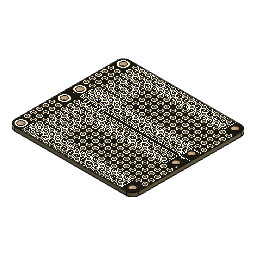
2890 Doubler FeatherWing (Autodesk Fusion 360 design; units mm, degrees)
part number: FEATHERWING_NODIM
Autodesk Fusion 360 part; units mm, degrees
sketch "sketch 305" plane through (0, 0, 0) normal (0, 0, 1) x (1, 0, 0)
  line L0 (2.54, 46.99) -> (48.26, 46.99)
  arc A0 (50.8, 44.45) -> (48.26, 46.99) centre (48.26, 44.45) ccw
  line L1 (50.8, 44.45) -> (50.8, 2.54)
  arc A1 (48.26, 0) -> (50.8, 2.54) centre (48.26, 2.54) ccw
  line L2 (48.26, 0) -> (2.54, 0)
  arc A2 (0, 2.54) -> (2.54, 0) centre (2.54, 2.54) ccw
  line L3 (0, 2.54) -> (0, 44.45)
  arc A3 (2.54, 46.99) -> (0, 44.45) centre (2.54, 44.45) ccw
extrude "Board" add sketch "sketch 305" along normal blind 1.57 makes body 1 in component "Board"
sketch "sketch 2573" plane through (0, 0, 0) normal (0, 0, 1) x (1, 0, 0)
  line L0 (0, 0) -> (50.8, 0)
  line L1 (50.8, 0) -> (50.8, 22.86)
  line L2 (50.8, 22.86) -> (0, 22.86)
  line L3 (0, 22.86) -> (0, 0)
extrude "FEATHERWING_DIM" add sketch "sketch 2573" along normal blind 0.1 separate body makes body 2 in component "FEATHERWING_DIM"
sketch "sketch 2713" plane through (0, 0, 0) normal (0, 0, 1) x (1, 0, 0)
  line L0 (-19.55, -0.5) -> (19.55, -0.5)
  line L1 (19.55, -0.5) -> (19.55, 0.5)
  line L2 (19.55, 0.5) -> (-19.55, 0.5)
  line L3 (-19.55, 0.5) -> (-19.55, -0.5)
extrude "1X16_ROUND_76MIL" add sketch "sketch 2713" along normal blind 0.1 separate body makes body 3 in component "1X16_ROUND_76MIL"
sketch "sketch 2853" plane through (0, 0, 0) normal (0, 0, 1) x (1, 0, 0)
  line L0 (-15.24, -0.635) -> (14.47, -0.635)
  line L1 (14.47, -0.635) -> (14.47, 0.635)
  line L2 (14.47, 0.635) -> (-15.24, 0.635)
  line L3 (-15.24, 0.635) -> (-15.24, -0.635)
extrude "1X12_ROUND_76MIL" add sketch "sketch 2853" along normal blind 0.1 separate body makes body 4 in component "1X12_ROUND_76MIL"
sketch "sketch 437" plane through (0, 0, 0) normal (0, 0, 1) x (1, 0, 0)
  circle A0 centre (13.97, 6.35) radius 0.55
  circle A1 centre (13.97, 8.89) radius 0.55
  circle A2 centre (13.97, 11.43) radius 0.55
  circle A3 centre (13.97, 13.97) radius 0.55
  circle A4 centre (13.97, 16.51) radius 0.55
  circle A5 centre (13.97, 19.05) radius 0.55
  circle A6 centre (13.97, 21.59) radius 0.55
  circle A7 centre (13.97, 45.72) radius 0.55
  circle A8 centre (13.97, 43.18) radius 0.55
  circle A9 centre (13.97, 40.64) radius 0.55
  circle A10 centre (13.97, 38.1) radius 0.55
  circle A11 centre (13.97, 35.56) radius 0.55
  circle A12 centre (13.97, 33.02) radius 0.55
  circle A13 centre (13.97, 30.48) radius 0.55
  circle A14 centre (8.89, 6.35) radius 0.55
  circle A15 centre (8.89, 8.89) radius 0.55
  circle A16 centre (8.89, 11.43) radius 0.55
  circle A17 centre (8.89, 13.97) radius 0.55
  circle A18 centre (8.89, 16.51) radius 0.55
  circle A19 centre (8.89, 19.05) radius 0.55
  circle A20 centre (8.89, 21.59) radius 0.55
  circle A21 centre (8.89, 30.48) radius 0.55
  circle A22 centre (8.89, 33.02) radius 0.55
  circle A23 centre (8.89, 35.56) radius 0.55
  circle A24 centre (8.89, 38.1) radius 0.55
  circle A25 centre (8.89, 40.64) radius 0.55
  circle A26 centre (8.89, 43.18) radius 0.55
  circle A27 centre (8.89, 45.72) radius 0.55
  circle A28 centre (6.35, 6.35) radius 0.55
  circle A29 centre (11.43, 6.35) radius 0.55
  circle A30 centre (11.43, 8.89) radius 0.55
  circle A31 centre (6.35, 8.89) radius 0.55
  circle A32 centre (6.35, 11.43) radius 0.55
  circle A33 centre (3.81, 6.35) radius 0.55
  circle A34 centre (1.27, 6.35) radius 0.55
  circle A35 centre (1.27, 8.89) radius 0.55
  circle A36 centre (3.81, 8.89) radius 0.55
  circle A37 centre (3.81, 11.43) radius 0.55
  circle A38 centre (1.27, 11.43) radius 0.55
  circle A39 centre (1.27, 13.97) radius 0.55
  circle A40 centre (3.81, 13.97) radius 0.55
  circle A41 centre (6.35, 13.97) radius 0.55
  circle A42 centre (11.43, 13.97) radius 0.55
  circle A43 centre (11.43, 11.43) radius 0.55
  circle A44 centre (1.27, 16.51) radius 0.55
  circle A45 centre (3.81, 16.51) radius 0.55
  circle A46 centre (6.35, 16.51) radius 0.55
  circle A47 centre (11.43, 16.51) radius 0.55
  circle A48 centre (11.43, 21.59) radius 0.55
  circle A49 centre (11.43, 19.05) radius 0.55
  circle A50 centre (6.35, 21.59) radius 0.55
  circle A51 centre (6.35, 19.05) radius 0.55
  circle A52 centre (16.51, 6.35) radius 0.55
  circle A53 centre (16.51, 8.89) radius 0.55
  circle A54 centre (16.51, 11.43) radius 0.55
  circle A55 centre (16.51, 13.97) radius 0.55
  circle A56 centre (16.51, 16.51) radius 0.55
  circle A57 centre (19.05, 16.51) radius 0.55
  circle A58 centre (19.05, 13.97) radius 0.55
  circle A59 centre (19.05, 11.43) radius 0.55
  circle A60 centre (19.05, 8.89) radius 0.55
  circle A61 centre (19.05, 6.35) radius 0.55
  circle A62 centre (21.59, 6.35) radius 0.55
  circle A63 centre (21.59, 8.89) radius 0.55
  circle A64 centre (21.59, 11.43) radius 0.55
  circle A65 centre (21.59, 13.97) radius 0.55
  circle A66 centre (21.59, 16.51) radius 0.55
  circle A67 centre (24.13, 16.51) radius 0.55
  circle A68 centre (24.13, 13.97) radius 0.55
  circle A69 centre (24.13, 11.43) radius 0.55
  circle A70 centre (24.13, 8.89) radius 0.55
  circle A71 centre (24.13, 6.35) radius 0.55
  circle A72 centre (26.67, 6.35) radius 0.55
  circle A73 centre (26.67, 8.89) radius 0.55
  circle A74 centre (26.67, 11.43) radius 0.55
  circle A75 centre (26.67, 13.97) radius 0.55
  circle A76 centre (26.67, 16.51) radius 0.55
  circle A77 centre (29.21, 16.51) radius 0.55
  circle A78 centre (29.21, 13.97) radius 0.55
  circle A79 centre (29.21, 11.43) radius 0.55
  circle A80 centre (29.21, 8.89) radius 0.55
  circle A81 centre (29.21, 6.35) radius 0.55
  circle A82 centre (31.75, 6.35) radius 0.55
  circle A83 centre (34.29, 6.35) radius 0.55
  circle A84 centre (36.83, 6.35) radius 0.55
  circle A85 centre (39.37, 6.35) radius 0.55
  circle A86 centre (41.91, 6.35) radius 0.55
  circle A87 centre (41.91, 8.89) radius 0.55
  circle A88 centre (41.91, 11.43) radius 0.55
  circle A89 centre (41.91, 13.97) radius 0.55
  circle A90 centre (41.91, 16.51) radius 0.55
  circle A91 centre (39.37, 16.51) radius 0.55
  circle A92 centre (39.37, 13.97) radius 0.55
  circle A93 centre (39.37, 11.43) radius 0.55
  circle A94 centre (39.37, 8.89) radius 0.55
  circle A95 centre (36.83, 8.89) radius 0.55
  circle A96 centre (36.83, 11.43) radius 0.55
  circle A97 centre (36.83, 13.97) radius 0.55
  circle A98 centre (36.83, 16.51) radius 0.55
  circle A99 centre (34.29, 16.51) radius 0.55
  circle A100 centre (34.29, 13.97) radius 0.55
  circle A101 centre (34.29, 11.43) radius 0.55
  circle A102 centre (34.29, 8.89) radius 0.55
  circle A103 centre (31.75, 8.89) radius 0.55
  circle A104 centre (31.75, 11.43) radius 0.55
  circle A105 centre (31.75, 13.97) radius 0.55
  circle A106 centre (31.75, 16.51) radius 0.55
  circle A107 centre (44.45, 16.51) radius 0.55
  circle A108 centre (44.45, 13.97) radius 0.55
  circle A109 centre (44.45, 11.43) radius 0.55
  circle A110 centre (44.45, 8.89) radius 0.55
  circle A111 centre (44.45, 6.35) radius 0.55
  circle A112 centre (46.99, 6.35) radius 0.55
  circle A113 centre (49.53, 6.35) radius 0.55
  circle A114 centre (49.53, 8.89) radius 0.55
  circle A115 centre (46.99, 8.89) radius 0.55
  circle A116 centre (46.99, 11.43) radius 0.55
  circle A117 centre (49.53, 11.43) radius 0.55
  circle A118 centre (49.53, 13.97) radius 0.55
  circle A119 centre (46.99, 13.97) radius 0.55
  circle A120 centre (46.99, 16.51) radius 0.55
  circle A121 centre (49.53, 16.51) radius 0.55
  circle A122 centre (44.45, 30.48) radius 0.55
  circle A123 centre (44.45, 33.02) radius 0.55
  circle A124 centre (44.45, 35.56) radius 0.55
  circle A125 centre (44.45, 38.1) radius 0.55
  circle A126 centre (44.45, 40.64) radius 0.55
  circle A127 centre (41.91, 40.64) radius 0.55
  circle A128 centre (41.91, 38.1) radius 0.55
  circle A129 centre (41.91, 35.56) radius 0.55
  circle A130 centre (41.91, 33.02) radius 0.55
  circle A131 centre (41.91, 30.48) radius 0.55
  circle A132 centre (46.99, 30.48) radius 0.55
  circle A133 centre (46.99, 33.02) radius 0.55
  circle A134 centre (46.99, 35.56) radius 0.55
  circle A135 centre (46.99, 38.1) radius 0.55
  circle A136 centre (46.99, 40.64) radius 0.55
  circle A137 centre (49.53, 40.64) radius 0.55
  circle A138 centre (49.53, 38.1) radius 0.55
  circle A139 centre (49.53, 35.56) radius 0.55
  circle A140 centre (49.53, 33.02) radius 0.55
  circle A141 centre (49.53, 30.48) radius 0.55
  circle A142 centre (39.37, 30.48) radius 0.55
  circle A143 centre (39.37, 33.02) radius 0.55
  circle A144 centre (39.37, 35.56) radius 0.55
  circle A145 centre (39.37, 38.1) radius 0.55
  circle A146 centre (39.37, 40.64) radius 0.55
  circle A147 centre (36.83, 40.64) radius 0.55
  circle A148 centre (36.83, 38.1) radius 0.55
  circle A149 centre (36.83, 35.56) radius 0.55
  circle A150 centre (36.83, 33.02) radius 0.55
  circle A151 centre (36.83, 30.48) radius 0.55
  circle A152 centre (34.29, 30.48) radius 0.55
  circle A153 centre (34.29, 33.02) radius 0.55
  circle A154 centre (34.29, 35.56) radius 0.55
  circle A155 centre (34.29, 38.1) radius 0.55
  circle A156 centre (34.29, 40.64) radius 0.55
  circle A157 centre (31.75, 40.64) radius 0.55
  circle A158 centre (31.75, 38.1) radius 0.55
  circle A159 centre (31.75, 35.56) radius 0.55
  circle A160 centre (31.75, 33.02) radius 0.55
  circle A161 centre (31.75, 30.48) radius 0.55
  circle A162 centre (29.21, 30.48) radius 0.55
  circle A163 centre (29.21, 33.02) radius 0.55
  circle A164 centre (29.21, 35.56) radius 0.55
  circle A165 centre (29.21, 38.1) radius 0.55
  circle A166 centre (29.21, 40.64) radius 0.55
  circle A167 centre (26.67, 40.64) radius 0.55
  circle A168 centre (26.67, 38.1) radius 0.55
  circle A169 centre (26.67, 35.56) radius 0.55
  circle A170 centre (26.67, 33.02) radius 0.55
  circle A171 centre (26.67, 30.48) radius 0.55
  circle A172 centre (24.13, 30.48) radius 0.55
  circle A173 centre (24.13, 33.02) radius 0.55
  circle A174 centre (24.13, 35.56) radius 0.55
  circle A175 centre (24.13, 38.1) radius 0.55
  circle A176 centre (24.13, 40.64) radius 0.55
  circle A177 centre (21.59, 40.64) radius 0.55
  circle A178 centre (21.59, 38.1) radius 0.55
  circle A179 centre (21.59, 35.56) radius 0.55
  circle A180 centre (21.59, 33.02) radius 0.55
  circle A181 centre (21.59, 30.48) radius 0.55
  circle A182 centre (19.05, 30.48) radius 0.55
  circle A183 centre (19.05, 33.02) radius 0.55
  circle A184 centre (19.05, 35.56) radius 0.55
  circle A185 centre (19.05, 38.1) radius 0.55
  circle A186 centre (19.05, 40.64) radius 0.55
  circle A187 centre (16.51, 40.64) radius 0.55
  circle A188 centre (16.51, 38.1) radius 0.55
  circle A189 centre (16.51, 35.56) radius 0.55
  circle A190 centre (16.51, 33.02) radius 0.55
  circle A191 centre (16.51, 30.48) radius 0.55
  circle A192 centre (11.43, 30.48) radius 0.55
  circle A193 centre (11.43, 33.02) radius 0.55
  circle A194 centre (11.43, 35.56) radius 0.55
  circle A195 centre (11.43, 38.1) radius 0.55
  circle A196 centre (11.43, 40.64) radius 0.55
  circle A197 centre (11.43, 43.18) radius 0.55
  circle A198 centre (11.43, 45.72) radius 0.55
  circle A199 centre (6.35, 30.48) radius 0.55
  circle A200 centre (6.35, 33.02) radius 0.55
  circle A201 centre (6.35, 35.56) radius 0.55
  circle A202 centre (6.35, 38.1) radius 0.55
  circle A203 centre (6.35, 40.64) radius 0.55
  circle A204 centre (6.35, 43.18) radius 0.55
  circle A205 centre (6.35, 45.72) radius 0.55
  circle A206 centre (3.81, 40.64) radius 0.55
  circle A207 centre (1.27, 40.64) radius 0.55
  circle A208 centre (1.27, 38.1) radius 0.55
  circle A209 centre (3.81, 38.1) radius 0.55
  circle A210 centre (3.81, 35.56) radius 0.55
  circle A211 centre (1.27, 35.56) radius 0.55
  circle A212 centre (1.27, 33.02) radius 0.55
  circle A213 centre (3.81, 33.02) radius 0.55
  circle A214 centre (3.81, 30.48) radius 0.55
  circle A215 centre (1.27, 30.48) radius 0.55
  circle A216 centre (48.26, 20.32) radius 1.27
  circle A217 centre (48.26, 2.54) radius 1.27
  circle A218 centre (2.54, 20.32) radius 1.25
  circle A219 centre (2.54, 2.54) radius 1.25
  circle A220 centre (16.51, 21.59) radius 0.5
  circle A221 centre (19.05, 21.59) radius 0.5
  circle A222 centre (21.59, 21.59) radius 0.5
  circle A223 centre (24.13, 21.59) radius 0.5
  circle A224 centre (26.67, 21.59) radius 0.5
  circle A225 centre (29.21, 21.59) radius 0.5
  circle A226 centre (31.75, 21.59) radius 0.5
  circle A227 centre (34.29, 21.59) radius 0.5
  circle A228 centre (36.83, 21.59) radius 0.5
  circle A229 centre (39.37, 21.59) radius 0.5
  circle A230 centre (41.91, 21.59) radius 0.5
  circle A231 centre (44.45, 21.59) radius 0.5
  circle A232 centre (16.51, 1.27) radius 0.5
  circle A233 centre (19.05, 1.27) radius 0.5
  circle A234 centre (21.59, 1.27) radius 0.5
  circle A235 centre (24.13, 1.27) radius 0.5
  circle A236 centre (26.67, 1.27) radius 0.5
  circle A237 centre (29.21, 1.27) radius 0.5
  circle A238 centre (31.75, 1.27) radius 0.5
  circle A239 centre (34.29, 1.27) radius 0.5
  circle A240 centre (36.83, 1.27) radius 0.5
  circle A241 centre (39.37, 1.27) radius 0.5
  circle A242 centre (41.91, 1.27) radius 0.5
  circle A243 centre (44.45, 1.27) radius 0.5
  circle A244 centre (13.97, 1.27) radius 0.5
  circle A245 centre (11.43, 1.27) radius 0.5
  circle A246 centre (8.89, 1.27) radius 0.5
  circle A247 centre (6.35, 1.27) radius 0.5
  circle A248 centre (48.26, 44.45) radius 1.27
  circle A249 centre (48.26, 26.67) radius 1.27
  circle A250 centre (2.54, 44.45) radius 1.25
  circle A251 centre (2.54, 26.67) radius 1.25
  circle A252 centre (16.51, 45.72) radius 0.5
  circle A253 centre (19.05, 45.72) radius 0.5
  circle A254 centre (21.59, 45.72) radius 0.5
  circle A255 centre (24.13, 45.72) radius 0.5
  circle A256 centre (26.67, 45.72) radius 0.5
  circle A257 centre (29.21, 45.72) radius 0.5
  circle A258 centre (31.75, 45.72) radius 0.5
  circle A259 centre (34.29, 45.72) radius 0.5
  circle A260 centre (36.83, 45.72) radius 0.5
  circle A261 centre (39.37, 45.72) radius 0.5
  circle A262 centre (41.91, 45.72) radius 0.5
  circle A263 centre (44.45, 45.72) radius 0.5
  circle A264 centre (16.51, 25.4) radius 0.5
  circle A265 centre (19.05, 25.4) radius 0.5
  circle A266 centre (21.59, 25.4) radius 0.5
  circle A267 centre (24.13, 25.4) radius 0.5
  circle A268 centre (26.67, 25.4) radius 0.5
  circle A269 centre (29.21, 25.4) radius 0.5
  circle A270 centre (31.75, 25.4) radius 0.5
  circle A271 centre (34.29, 25.4) radius 0.5
  circle A272 centre (36.83, 25.4) radius 0.5
  circle A273 centre (39.37, 25.4) radius 0.5
  circle A274 centre (41.91, 25.4) radius 0.5
  circle A275 centre (44.45, 25.4) radius 0.5
  circle A276 centre (13.97, 25.4) radius 0.5
  circle A277 centre (11.43, 25.4) radius 0.5
  circle A278 centre (8.89, 25.4) radius 0.5
  circle A279 centre (6.35, 25.4) radius 0.5
  circle A280 centre (44.45, 3.81) radius 0.5
  circle A281 centre (41.91, 3.81) radius 0.5
  circle A282 centre (39.37, 3.81) radius 0.5
  circle A283 centre (36.83, 3.81) radius 0.5
  circle A284 centre (34.29, 3.81) radius 0.5
  circle A285 centre (31.75, 3.81) radius 0.5
  circle A286 centre (29.21, 3.81) radius 0.5
  circle A287 centre (26.67, 3.81) radius 0.5
  circle A288 centre (24.13, 3.81) radius 0.5
  circle A289 centre (21.59, 3.81) radius 0.5
  circle A290 centre (19.05, 3.81) radius 0.5
  circle A291 centre (16.51, 3.81) radius 0.5
  circle A292 centre (13.97, 3.81) radius 0.5
  circle A293 centre (11.43, 3.81) radius 0.5
  circle A294 centre (8.89, 3.81) radius 0.5
  circle A295 centre (6.35, 3.81) radius 0.5
  circle A296 centre (44.45, 27.94) radius 0.5
  circle A297 centre (41.91, 27.94) radius 0.5
  circle A298 centre (39.37, 27.94) radius 0.5
  circle A299 centre (36.83, 27.94) radius 0.5
  circle A300 centre (34.29, 27.94) radius 0.5
  circle A301 centre (31.75, 27.94) radius 0.5
  circle A302 centre (29.21, 27.94) radius 0.5
  circle A303 centre (26.67, 27.94) radius 0.5
  circle A304 centre (24.13, 27.94) radius 0.5
  circle A305 centre (21.59, 27.94) radius 0.5
  circle A306 centre (19.05, 27.94) radius 0.5
  circle A307 centre (16.51, 27.94) radius 0.5
  circle A308 centre (13.97, 27.94) radius 0.5
  circle A309 centre (11.43, 27.94) radius 0.5
  circle A310 centre (8.89, 27.94) radius 0.5
  circle A311 centre (6.35, 27.94) radius 0.5
  circle A312 centre (16.51, 19.05) radius 0.5
  circle A313 centre (19.05, 19.05) radius 0.5
  circle A314 centre (21.59, 19.05) radius 0.5
  circle A315 centre (24.13, 19.05) radius 0.5
  circle A316 centre (26.67, 19.05) radius 0.5
  circle A317 centre (29.21, 19.05) radius 0.5
  circle A318 centre (31.75, 19.05) radius 0.5
  circle A319 centre (34.29, 19.05) radius 0.5
  circle A320 centre (36.83, 19.05) radius 0.5
  circle A321 centre (39.37, 19.05) radius 0.5
  circle A322 centre (41.91, 19.05) radius 0.5
  circle A323 centre (44.45, 19.05) radius 0.5
  circle A324 centre (16.51, 43.18) radius 0.5
  circle A325 centre (19.05, 43.18) radius 0.5
  circle A326 centre (21.59, 43.18) radius 0.5
  circle A327 centre (24.13, 43.18) radius 0.5
  circle A328 centre (26.67, 43.18) radius 0.5
  circle A329 centre (29.21, 43.18) radius 0.5
  circle A330 centre (31.75, 43.18) radius 0.5
  circle A331 centre (34.29, 43.18) radius 0.5
  circle A332 centre (36.83, 43.18) radius 0.5
  circle A333 centre (39.37, 43.18) radius 0.5
  circle A334 centre (41.91, 43.18) radius 0.5
  circle A335 centre (44.45, 43.18) radius 0.5
extrude "Extrude2" cut sketch "sketch 437" along normal blind 1.57 bodies 1 in component "Board"
component "PCB Component" placed x (1, 0, 0) y (0, 1, 0) z (0, 0, 1) at (0, 0, 0)
component "Board" placed x (1, 0, 0) y (0, 1, 0) z (0, 0, 1) at (0, 0, 0) in component "PCB Component"
component "FEATHERWING_DIM" placed x (1, 0, 0) y (0, 1, 0) z (0, 0, 1) at (0, 0, 1.57) in component "PCB Component"
component "FEATHERWING_DIM" placed x (1, 0, 0) y (0, 1, 0) z (0, 0, 1) at (0, 24.13, 1.57) in component "PCB Component"
component "1X16_ROUND_76MIL" placed x (-1, 0, 0) y (0, -1, 0) z (0, 0, 1) at (25.4, 3.81, 1.57) in component "PCB Component"
component "1X16_ROUND_76MIL" placed x (-1, 0, 0) y (0, -1, 0) z (0, 0, 1) at (25.4, 27.94, 1.57) in component "PCB Component"
component "1X12_ROUND_76MIL" placed x (1, 0, 0) y (0, 1, 0) z (0, 0, 1) at (30.48, 19.05, 1.57) in component "PCB Component"
component "1X12_ROUND_76MIL" placed x (1, 0, 0) y (0, 1, 0) z (0, 0, 1) at (30.48, 43.18, 1.57) in component "PCB Component"
named bodies: "Board", "FEATHERWING_DIM", "1X16_ROUND_76MIL", "1X12_ROUND_76MIL"
